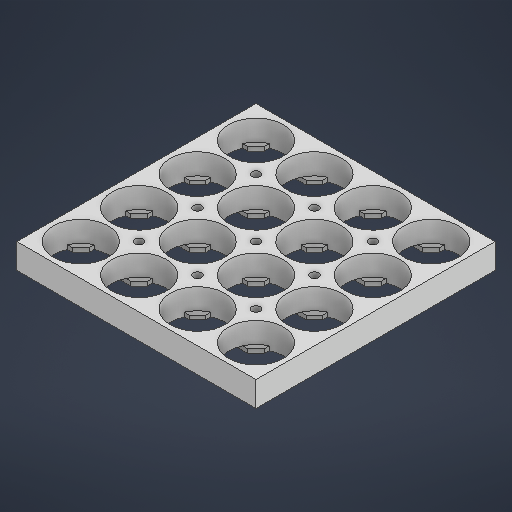
# Autodesk Inventor part: battery_pack_16s_rear
Saved by Autodesk Inventor 2026.1 (Build 301233000, 233)
## iProperties
Created: 2026-03-08
Part Number: battery_pack_16s_rear
Material: Generic
Document SubType Name: Modeling
Designer: aaron
Density: 1 g/cm^3
Appearance: Default
Author: aaron
Autodesk Inventor part; units mm, degrees
ref_plane "YZ Plane" through (0, 0, 0) normal (1, 0, 0) x (0, 1, 0)
ref_plane "XZ Plane" through (0, 0, 0) normal (0, 1, 0) x (-1, 0, 0)
ref_plane "XY Plane" through (0, 0, 0) normal (0, 0, 1) x (1, 0, 0)
sketch "Sketch1" plane through (0, 0, 0) normal (0, 1, 0) x (-1, 0, 0)
  circle A0 centre (10.0499, 9.6753) radius 13.1
  line L0 (10.0499, 9.6753) -> (10.0499, 15.7412)
  line L1 (10.0499, 9.6753) -> (16.8689, 9.6753)
  circle A1 centre (10.0499, 37.6753) radius 13.1
  circle A2 centre (10.0499, 65.6753) radius 13.1
  circle A3 centre (10.0499, 93.6753) radius 13.1
  circle A4 centre (38.0499, 9.6753) radius 13.1
  circle A5 centre (38.0499, 37.6753) radius 13.1
  circle A6 centre (38.0499, 65.6753) radius 13.1
  circle A7 centre (38.0499, 93.6753) radius 13.1
  circle A8 centre (66.0499, 9.6753) radius 13.1
  circle A9 centre (66.0499, 37.6753) radius 13.1
  circle A10 centre (66.0499, 65.6753) radius 13.1
  circle A11 centre (66.0499, 93.6753) radius 13.1
  circle A12 centre (94.0499, 9.6753) radius 13.1
  circle A13 centre (94.0499, 37.6753) radius 13.1
  circle A14 centre (94.0499, 65.6753) radius 13.1
  circle A15 centre (94.0499, 93.6753) radius 13.1
  line L2 (109.3499, 108.9753) -> (-5.2501, 108.9753)
  line L3 (-5.2501, 108.9753) -> (-5.2501, -5.6247)
  line L4 (-5.2501, -5.6247) -> (109.3499, -5.6247)
  line L5 (109.3499, -5.6247) -> (109.3499, 108.9753)
  point P0 (0, 0)
  dimension "d0" = 26.2
  dimension "d3" = 28
  dimension "d6" = 28
  dimension "d9" = 15.3
  dimension "d10" = 15.3
  dimension "d11" = 15.3
  dimension "d12" = 15.3
  constraints: 16 centre point, 12 end point, 3 horizontal, 2 parallel, 2 vertical, 1 perpendicular, 30 other
  measures "d0" diameter of A0
  measures "d3" distance of L0.start A1.centre
  measures "d6" distance of L0.start A4.centre
  measures "d9" distance from line of L5 A15.centre
  measures "d10" distance from line of L3 A3.centre
  measures "d11" distance from line of L2 A15.centre
  measures "d12" distance from line of L4 A12.centre
extrude "Extrusion1" add sketch "Sketch1" along normal blind 10
sketch "Sketch2" plane through (0, 0, 0) normal (0, -1, 0) x (1, 0, 0)
  line L0 (-109.3499, 108.9753) -> (5.2501, 108.9753) projected
  line L1 (5.2501, 108.9753) -> (5.2501, -5.6247) projected
  line L2 (5.2501, -5.6247) -> (-109.3499, -5.6247) projected
  line L3 (-109.3499, -5.6247) -> (-109.3499, 108.9753) projected
  circle A0 centre (-10.0499, 93.6753) radius 13.1 projected
  circle A1 centre (-10.0499, 9.6753) radius 13.1 projected
  line L4 (8.4501, 116.1753) -> (-0.5499, 116.1753)
  line L5 (-4.5499, 112.1753) -> (-4.5499, 103.1753)
  line L6 (-0.5499, 99.1753) -> (8.4501, 99.1753)
  line L7 (12.4501, 103.1753) -> (12.4501, 112.1753)
  line L8 (-10.0499, 93.6753) -> (15.9741, 93.6753)
  line L9 (-10.0499, 93.6753) -> (-10.0499, 119.9276)
  circle A2 centre (-38.0499, 93.6753) radius 13.1 projected
  circle A3 centre (-38.0499, 65.6753) radius 13.1 projected
  line L10 (-38.0499, 93.6753) -> (-38.0499, 65.6753)
  circle A4 centre (-66.0499, 65.6753) radius 13.1 projected
  line L11 (-38.0499, 65.6753) -> (-66.0499, 65.6753)
  line L12 (-4.5499, 103.1753) -> (-0.5499, 99.1753)
  line L13 (-0.5499, 116.1753) -> (-4.5499, 112.1753)
  line L14 (8.4501, 116.1753) -> (12.4501, 112.1753)
  line L15 (8.4501, 99.1753) -> (12.4501, 103.1753)
  line L16 (8.4501, 88.1753) -> (12.4501, 84.1753)
  line L17 (12.4501, 75.1753) -> (12.4501, 84.1753)
  line L18 (8.4501, 88.1753) -> (-0.5499, 88.1753)
  line L19 (-0.5499, 88.1753) -> (-4.5499, 84.1753)
  line L20 (-4.5499, 84.1753) -> (-4.5499, 75.1753)
  line L21 (-4.5499, 75.1753) -> (-0.5499, 71.1753)
  line L22 (-0.5499, 71.1753) -> (8.4501, 71.1753)
  line L23 (8.4501, 71.1753) -> (12.4501, 75.1753)
  line L24 (8.4501, 60.1753) -> (12.4501, 56.1753)
  line L25 (12.4501, 47.1753) -> (12.4501, 56.1753)
  line L26 (8.4501, 60.1753) -> (-0.5499, 60.1753)
  line L27 (-0.5499, 60.1753) -> (-4.5499, 56.1753)
  line L28 (-4.5499, 56.1753) -> (-4.5499, 47.1753)
  line L29 (-4.5499, 47.1753) -> (-0.5499, 43.1753)
  line L30 (-0.5499, 43.1753) -> (8.4501, 43.1753)
  line L31 (8.4501, 43.1753) -> (12.4501, 47.1753)
  line L32 (8.4501, 32.1753) -> (12.4501, 28.1753)
  line L33 (12.4501, 19.1753) -> (12.4501, 28.1753)
  line L34 (8.4501, 32.1753) -> (-0.5499, 32.1753)
  line L35 (-0.5499, 32.1753) -> (-4.5499, 28.1753)
  line L36 (-4.5499, 28.1753) -> (-4.5499, 19.1753)
  line L37 (-4.5499, 19.1753) -> (-0.5499, 15.1753)
  line L38 (-0.5499, 15.1753) -> (8.4501, 15.1753)
  line L39 (8.4501, 15.1753) -> (12.4501, 19.1753)
  line L40 (8.4501, 4.1753) -> (12.4501, 0.1753)
  line L41 (12.4501, -8.8247) -> (12.4501, 0.1753)
  line L42 (8.4501, 4.1753) -> (-0.5499, 4.1753)
  line L43 (-0.5499, 4.1753) -> (-4.5499, 0.1753)
  line L44 (-4.5499, 0.1753) -> (-4.5499, -8.8247)
  line L45 (-4.5499, -8.8247) -> (-0.5499, -12.8247)
  line L46 (-0.5499, -12.8247) -> (8.4501, -12.8247)
  line L47 (8.4501, -12.8247) -> (12.4501, -8.8247)
  line L48 (-19.5499, 116.1753) -> (-15.5499, 112.1753)
  line L49 (-15.5499, 103.1753) -> (-15.5499, 112.1753)
  line L50 (-19.5499, 116.1753) -> (-28.5499, 116.1753)
  line L51 (-28.5499, 116.1753) -> (-32.5499, 112.1753)
  line L52 (-32.5499, 112.1753) -> (-32.5499, 103.1753)
  line L53 (-32.5499, 103.1753) -> (-28.5499, 99.1753)
  line L54 (-28.5499, 99.1753) -> (-19.5499, 99.1753)
  line L55 (-19.5499, 99.1753) -> (-15.5499, 103.1753)
  line L56 (-19.5499, 88.1753) -> (-15.5499, 84.1753)
  line L57 (-15.5499, 75.1753) -> (-15.5499, 84.1753)
  line L58 (-19.5499, 88.1753) -> (-28.5499, 88.1753)
  line L59 (-28.5499, 88.1753) -> (-32.5499, 84.1753)
  line L60 (-32.5499, 84.1753) -> (-32.5499, 75.1753)
  line L61 (-32.5499, 75.1753) -> (-28.5499, 71.1753)
  line L62 (-28.5499, 71.1753) -> (-19.5499, 71.1753)
  line L63 (-19.5499, 71.1753) -> (-15.5499, 75.1753)
  line L64 (-19.5499, 60.1753) -> (-15.5499, 56.1753)
  line L65 (-15.5499, 47.1753) -> (-15.5499, 56.1753)
  line L66 (-19.5499, 60.1753) -> (-28.5499, 60.1753)
  line L67 (-28.5499, 60.1753) -> (-32.5499, 56.1753)
  line L68 (-32.5499, 56.1753) -> (-32.5499, 47.1753)
  line L69 (-32.5499, 47.1753) -> (-28.5499, 43.1753)
  line L70 (-28.5499, 43.1753) -> (-19.5499, 43.1753)
  line L71 (-19.5499, 43.1753) -> (-15.5499, 47.1753)
  line L72 (-19.5499, 32.1753) -> (-15.5499, 28.1753)
  line L73 (-15.5499, 19.1753) -> (-15.5499, 28.1753)
  line L74 (-19.5499, 32.1753) -> (-28.5499, 32.1753)
  line L75 (-28.5499, 32.1753) -> (-32.5499, 28.1753)
  line L76 (-32.5499, 28.1753) -> (-32.5499, 19.1753)
  line L77 (-32.5499, 19.1753) -> (-28.5499, 15.1753)
  line L78 (-28.5499, 15.1753) -> (-19.5499, 15.1753)
  line L79 (-19.5499, 15.1753) -> (-15.5499, 19.1753)
  line L80 (-19.5499, 4.1753) -> (-15.5499, 0.1753)
  line L81 (-15.5499, -8.8247) -> (-15.5499, 0.1753)
  line L82 (-19.5499, 4.1753) -> (-28.5499, 4.1753)
  line L83 (-28.5499, 4.1753) -> (-32.5499, 0.1753)
  line L84 (-32.5499, 0.1753) -> (-32.5499, -8.8247)
  line L85 (-32.5499, -8.8247) -> (-28.5499, -12.8247)
  line L86 (-28.5499, -12.8247) -> (-19.5499, -12.8247)
  line L87 (-19.5499, -12.8247) -> (-15.5499, -8.8247)
  line L88 (-47.5499, 116.1753) -> (-43.5499, 112.1753)
  line L89 (-43.5499, 103.1753) -> (-43.5499, 112.1753)
  line L90 (-47.5499, 116.1753) -> (-56.5499, 116.1753)
  line L91 (-56.5499, 116.1753) -> (-60.5499, 112.1753)
  line L92 (-60.5499, 112.1753) -> (-60.5499, 103.1753)
  line L93 (-60.5499, 103.1753) -> (-56.5499, 99.1753)
  line L94 (-56.5499, 99.1753) -> (-47.5499, 99.1753)
  line L95 (-47.5499, 99.1753) -> (-43.5499, 103.1753)
  line L96 (-47.5499, 88.1753) -> (-43.5499, 84.1753)
  line L97 (-43.5499, 75.1753) -> (-43.5499, 84.1753)
  line L98 (-47.5499, 88.1753) -> (-56.5499, 88.1753)
  line L99 (-56.5499, 88.1753) -> (-60.5499, 84.1753)
  line L100 (-60.5499, 84.1753) -> (-60.5499, 75.1753)
  line L101 (-60.5499, 75.1753) -> (-56.5499, 71.1753)
  line L102 (-56.5499, 71.1753) -> (-47.5499, 71.1753)
  line L103 (-47.5499, 71.1753) -> (-43.5499, 75.1753)
  line L104 (-47.5499, 60.1753) -> (-43.5499, 56.1753)
  line L105 (-43.5499, 47.1753) -> (-43.5499, 56.1753)
  line L106 (-47.5499, 60.1753) -> (-56.5499, 60.1753)
  line L107 (-56.5499, 60.1753) -> (-60.5499, 56.1753)
  line L108 (-60.5499, 56.1753) -> (-60.5499, 47.1753)
  line L109 (-60.5499, 47.1753) -> (-56.5499, 43.1753)
  line L110 (-56.5499, 43.1753) -> (-47.5499, 43.1753)
  line L111 (-47.5499, 43.1753) -> (-43.5499, 47.1753)
  line L112 (-47.5499, 32.1753) -> (-43.5499, 28.1753)
  line L113 (-43.5499, 19.1753) -> (-43.5499, 28.1753)
  line L114 (-47.5499, 32.1753) -> (-56.5499, 32.1753)
  line L115 (-56.5499, 32.1753) -> (-60.5499, 28.1753)
  line L116 (-60.5499, 28.1753) -> (-60.5499, 19.1753)
  line L117 (-60.5499, 19.1753) -> (-56.5499, 15.1753)
  line L118 (-56.5499, 15.1753) -> (-47.5499, 15.1753)
  line L119 (-47.5499, 15.1753) -> (-43.5499, 19.1753)
  line L120 (-47.5499, 4.1753) -> (-43.5499, 0.1753)
  line L121 (-43.5499, -8.8247) -> (-43.5499, 0.1753)
  line L122 (-47.5499, 4.1753) -> (-56.5499, 4.1753)
  line L123 (-56.5499, 4.1753) -> (-60.5499, 0.1753)
  line L124 (-60.5499, 0.1753) -> (-60.5499, -8.8247)
  line L125 (-60.5499, -8.8247) -> (-56.5499, -12.8247)
  line L126 (-56.5499, -12.8247) -> (-47.5499, -12.8247)
  line L127 (-47.5499, -12.8247) -> (-43.5499, -8.8247)
  line L128 (-75.5499, 116.1753) -> (-71.5499, 112.1753)
  line L129 (-71.5499, 103.1753) -> (-71.5499, 112.1753)
  line L130 (-75.5499, 116.1753) -> (-84.5499, 116.1753)
  line L131 (-84.5499, 116.1753) -> (-88.5499, 112.1753)
  line L132 (-88.5499, 112.1753) -> (-88.5499, 103.1753)
  line L133 (-88.5499, 103.1753) -> (-84.5499, 99.1753)
  line L134 (-84.5499, 99.1753) -> (-75.5499, 99.1753)
  line L135 (-75.5499, 99.1753) -> (-71.5499, 103.1753)
  line L136 (-75.5499, 88.1753) -> (-71.5499, 84.1753)
  line L137 (-71.5499, 75.1753) -> (-71.5499, 84.1753)
  line L138 (-75.5499, 88.1753) -> (-84.5499, 88.1753)
  line L139 (-84.5499, 88.1753) -> (-88.5499, 84.1753)
  line L140 (-88.5499, 84.1753) -> (-88.5499, 75.1753)
  line L141 (-88.5499, 75.1753) -> (-84.5499, 71.1753)
  line L142 (-84.5499, 71.1753) -> (-75.5499, 71.1753)
  line L143 (-75.5499, 71.1753) -> (-71.5499, 75.1753)
  line L144 (-75.5499, 60.1753) -> (-71.5499, 56.1753)
  line L145 (-71.5499, 47.1753) -> (-71.5499, 56.1753)
  line L146 (-75.5499, 60.1753) -> (-84.5499, 60.1753)
  line L147 (-84.5499, 60.1753) -> (-88.5499, 56.1753)
  line L148 (-88.5499, 56.1753) -> (-88.5499, 47.1753)
  line L149 (-88.5499, 47.1753) -> (-84.5499, 43.1753)
  line L150 (-84.5499, 43.1753) -> (-75.5499, 43.1753)
  line L151 (-75.5499, 43.1753) -> (-71.5499, 47.1753)
  line L152 (-75.5499, 32.1753) -> (-71.5499, 28.1753)
  line L153 (-71.5499, 19.1753) -> (-71.5499, 28.1753)
  line L154 (-75.5499, 32.1753) -> (-84.5499, 32.1753)
  line L155 (-84.5499, 32.1753) -> (-88.5499, 28.1753)
  line L156 (-88.5499, 28.1753) -> (-88.5499, 19.1753)
  line L157 (-88.5499, 19.1753) -> (-84.5499, 15.1753)
  line L158 (-84.5499, 15.1753) -> (-75.5499, 15.1753)
  line L159 (-75.5499, 15.1753) -> (-71.5499, 19.1753)
  line L160 (-75.5499, 4.1753) -> (-71.5499, 0.1753)
  line L161 (-71.5499, -8.8247) -> (-71.5499, 0.1753)
  line L162 (-75.5499, 4.1753) -> (-84.5499, 4.1753)
  line L163 (-84.5499, 4.1753) -> (-88.5499, 0.1753)
  line L164 (-88.5499, 0.1753) -> (-88.5499, -8.8247)
  line L165 (-88.5499, -8.8247) -> (-84.5499, -12.8247)
  line L166 (-84.5499, -12.8247) -> (-75.5499, -12.8247)
  line L167 (-75.5499, -12.8247) -> (-71.5499, -8.8247)
  line L168 (-103.5499, 116.1753) -> (-99.5499, 112.1753)
  line L169 (-99.5499, 103.1753) -> (-99.5499, 112.1753)
  line L170 (-103.5499, 116.1753) -> (-112.5499, 116.1753)
  line L171 (-112.5499, 116.1753) -> (-116.5499, 112.1753)
  line L172 (-116.5499, 112.1753) -> (-116.5499, 103.1753)
  line L173 (-116.5499, 103.1753) -> (-112.5499, 99.1753)
  line L174 (-112.5499, 99.1753) -> (-103.5499, 99.1753)
  line L175 (-103.5499, 99.1753) -> (-99.5499, 103.1753)
  line L176 (-103.5499, 88.1753) -> (-99.5499, 84.1753)
  line L177 (-99.5499, 75.1753) -> (-99.5499, 84.1753)
  line L178 (-103.5499, 88.1753) -> (-112.5499, 88.1753)
  line L179 (-112.5499, 88.1753) -> (-116.5499, 84.1753)
  line L180 (-116.5499, 84.1753) -> (-116.5499, 75.1753)
  line L181 (-116.5499, 75.1753) -> (-112.5499, 71.1753)
  line L182 (-112.5499, 71.1753) -> (-103.5499, 71.1753)
  line L183 (-103.5499, 71.1753) -> (-99.5499, 75.1753)
  line L184 (-103.5499, 60.1753) -> (-99.5499, 56.1753)
  line L185 (-99.5499, 47.1753) -> (-99.5499, 56.1753)
  line L186 (-103.5499, 60.1753) -> (-112.5499, 60.1753)
  line L187 (-112.5499, 60.1753) -> (-116.5499, 56.1753)
  line L188 (-116.5499, 56.1753) -> (-116.5499, 47.1753)
  line L189 (-116.5499, 47.1753) -> (-112.5499, 43.1753)
  line L190 (-112.5499, 43.1753) -> (-103.5499, 43.1753)
  line L191 (-103.5499, 43.1753) -> (-99.5499, 47.1753)
  line L192 (-103.5499, 32.1753) -> (-99.5499, 28.1753)
  line L193 (-99.5499, 19.1753) -> (-99.5499, 28.1753)
  line L194 (-103.5499, 32.1753) -> (-112.5499, 32.1753)
  line L195 (-112.5499, 32.1753) -> (-116.5499, 28.1753)
  line L196 (-116.5499, 28.1753) -> (-116.5499, 19.1753)
  line L197 (-116.5499, 19.1753) -> (-112.5499, 15.1753)
  line L198 (-112.5499, 15.1753) -> (-103.5499, 15.1753)
  line L199 (-103.5499, 15.1753) -> (-99.5499, 19.1753)
  line L200 (-103.5499, 4.1753) -> (-99.5499, 0.1753)
  line L201 (-99.5499, -8.8247) -> (-99.5499, 0.1753)
  line L202 (-103.5499, 4.1753) -> (-112.5499, 4.1753)
  line L203 (-112.5499, 4.1753) -> (-116.5499, 0.1753)
  line L204 (-116.5499, 0.1753) -> (-116.5499, -8.8247)
  line L205 (-116.5499, -8.8247) -> (-112.5499, -12.8247)
  line L206 (-112.5499, -12.8247) -> (-103.5499, -12.8247)
  line L207 (-103.5499, -12.8247) -> (-99.5499, -8.8247)
  circle A5 centre (-94.0499, 9.6753) radius 13.1 projected
  circle A6 centre (-94.0499, 37.6753) radius 13.1 projected
  circle A7 centre (-94.0499, 65.6753) radius 13.1 projected
  circle A8 centre (-94.0499, 93.6753) radius 13.1 projected
  circle A9 centre (-66.0499, 93.6753) radius 13.1 projected
  circle A10 centre (-66.0499, 37.6753) radius 13.1 projected
  circle A11 centre (-38.0499, 37.6753) radius 13.1 projected
  circle A12 centre (-66.0499, 9.6753) radius 13.1 projected
  circle A13 centre (-38.0499, 9.6753) radius 13.1 projected
  circle A14 centre (-10.0499, 37.6753) radius 13.1 projected
  circle A15 centre (-10.0499, 65.6753) radius 13.1 projected
  point P0 (12.4501, 116.1753)
  point P1 (-4.5499, 99.1753)
  point P2 (-4.5499, 116.1753)
  point P3 (12.4501, 99.1753)
  point P4 (-71.5499, -5.6247)
  point P5 (-77.9394, 4.1753)
  point P6 (-77.9394, 15.1753)
  point P7 (-71.5499, 21.5648)
  point P8 (-60.5499, 21.5648)
  point P9 (-54.1604, 15.1753)
  point P10 (-54.1604, 4.1753)
  point P11 (-60.5499, -5.6247)
  point P12 (1.8396, 99.1753)
  point P13 (1.8396, 88.1753)
  point P14 (-4.5499, 81.7858)
  point P15 (-15.5499, 81.7858)
  point P16 (-21.9394, 88.1753)
  point P17 (-21.9394, 99.1753)
  point P18 (-15.5499, 105.5648)
  point P19 (-4.5499, 105.5648)
  point P20 (1.8396, 4.1753)
  point P21 (-4.5499, -2.2142)
  point P22 (-15.5499, -2.2142)
  point P23 (-21.9394, 4.1753)
  point P24 (-21.9394, 15.1753)
  point P25 (-15.5499, 21.5648)
  point P26 (-4.5499, 21.5648)
  point P27 (1.8396, 15.1753)
  point P28 (-26.1604, 99.1753)
  point P29 (-26.1604, 88.1753)
  point P30 (-32.5499, 81.7858)
  point P31 (-43.5499, 81.7858)
  point P32 (-49.9394, 88.1753)
  point P33 (-49.9394, 99.1753)
  point P34 (-43.5499, 105.5648)
  point P35 (-32.5499, 105.5648)
  point P36 (-32.5499, 77.5648)
  point P37 (-26.1604, 71.1753)
  point P38 (-26.1604, 60.1753)
  point P39 (-32.5499, 53.7858)
  point P40 (-43.5499, 53.7858)
  point P41 (-49.9394, 60.1753)
  point P42 (-49.9394, 71.1753)
  point P43 (-43.5499, 77.5648)
  point P44 (-54.1604, 60.1753)
  point P45 (-60.5499, 53.7858)
  point P46 (-71.5499, 53.7858)
  point P47 (-77.9394, 60.1753)
  point P48 (-77.9394, 71.1753)
  point P49 (-71.5499, 77.5648)
  point P50 (-60.5499, 77.5648)
  point P51 (-54.1604, 71.1753)
  point P52 (-99.5499, -2.2142)
  point P53 (-105.9394, 4.1753)
  point P54 (-105.9394, 15.1753)
  point P55 (-99.5499, 21.5648)
  point P56 (-88.5499, 21.5648)
  point P57 (-82.1604, 15.1753)
  point P58 (-82.1604, 4.1753)
  point P59 (-88.5499, -2.2142)
  point P60 (-99.5499, 25.7858)
  point P61 (-105.9394, 32.1753)
  point P62 (-105.9394, 43.1753)
  point P63 (-99.5499, 49.5648)
  point P64 (-88.5499, 49.5648)
  point P65 (-82.1604, 43.1753)
  point P66 (-82.1604, 32.1753)
  point P67 (-88.5499, 25.7858)
  point P68 (-99.5499, 105.5648)
  point P69 (-88.5499, 105.5648)
  point P70 (-82.1604, 99.1753)
  point P71 (-82.1604, 88.1753)
  point P72 (-88.5499, 81.7858)
  point P73 (-99.5499, 81.7858)
  point P74 (-105.9394, 88.1753)
  point P75 (-105.9394, 99.1753)
  point P76 (-54.1604, 99.1753)
  point P77 (-54.1604, 88.1753)
  point P78 (-60.5499, 81.7858)
  point P79 (-71.5499, 81.7858)
  point P80 (-77.9394, 88.1753)
  point P81 (-77.9394, 99.1753)
  point P82 (-71.5499, 105.5648)
  point P83 (-60.5499, 105.5648)
  point P84 (-43.5499, 21.5648)
  point P85 (-32.5499, 21.5648)
  point P86 (-26.1604, 15.1753)
  point P87 (-26.1604, 4.1753)
  point P88 (-32.5499, -2.2142)
  point P89 (-43.5499, -2.2142)
  point P90 (-49.9394, 4.1753)
  point P91 (-49.9394, 15.1753)
  point P92 (1.8396, 71.1753)
  point P93 (1.8396, 60.1753)
  point P94 (-4.5499, 53.7858)
  point P95 (-15.5499, 53.7858)
  point P96 (-21.9394, 60.1753)
  point P97 (-21.9394, 71.1753)
  point P98 (-15.5499, 77.5648)
  point P99 (-4.5499, 77.5648)
  point P100 (1.8396, 32.1753)
  point P101 (-4.5499, 25.7858)
  point P102 (-15.5499, 25.7858)
  point P103 (-21.9394, 32.1753)
  point P104 (-21.9394, 43.1753)
  point P105 (-15.5499, 49.5648)
  point P106 (-4.5499, 49.5648)
  point P107 (1.8396, 43.1753)
  point P108 (-49.9394, 43.1753)
  point P109 (-43.5499, 49.5648)
  point P110 (-32.5499, 49.5648)
  point P111 (-26.1604, 43.1753)
  point P112 (-26.1604, 32.1753)
  point P113 (-32.5499, 25.7858)
  point P114 (-43.5499, 25.7858)
  point P115 (-49.9394, 32.1753)
  point P116 (-77.9394, 43.1753)
  point P117 (-71.5499, 49.5648)
  point P118 (-60.5499, 49.5648)
  point P119 (-54.1604, 43.1753)
  point P120 (-54.1604, 32.1753)
  point P121 (-60.5499, 25.7858)
  point P122 (-71.5499, 25.7858)
  point P123 (-77.9394, 32.1753)
  point P124 (-99.5499, 53.7858)
  point P125 (-105.9394, 60.1753)
  point P126 (-105.9394, 71.1753)
  point P127 (-99.5499, 77.5648)
  point P128 (-88.5499, 77.5648)
  point P129 (-82.1604, 71.1753)
  point P130 (-82.1604, 60.1753)
  point P131 (-88.5499, 53.7858)
  point P132 (-60.5499, -2.2142)
  point P133 (-71.5499, -2.2142)
  point P134 (5.2501, 99.1753)
  point P135 (-4.5499, 108.9753)
  point P136 (5.2501, 71.1753)
  point P137 (5.2501, 88.1753)
  point P138 (-109.3499, 4.1753)
  point P139 (-99.5499, -5.6247)
  point P140 (-109.3499, 32.1753)
  point P141 (-109.3499, 15.1753)
  point P142 (-109.3499, 60.1753)
  point P143 (-109.3499, 43.1753)
  point P144 (-99.5499, 108.9753)
  point P145 (-109.3499, 99.1753)
  point P146 (-109.3499, 88.1753)
  point P147 (-109.3499, 71.1753)
  point P148 (-88.5499, -5.6247)
  point P149 (-71.5499, 108.9753)
  point P150 (-88.5499, 108.9753)
  point P151 (-43.5499, -5.6247)
  point P152 (-43.5499, 108.9753)
  point P153 (-60.5499, 108.9753)
  point P154 (-4.5499, -5.6247)
  point P155 (5.2501, 4.1753)
  point P156 (-32.5499, -5.6247)
  point P157 (-15.5499, -5.6247)
  point P158 (5.2501, 15.1753)
  point P159 (5.2501, 32.1753)
  point P160 (5.2501, 43.1753)
  point P161 (5.2501, 60.1753)
  point P162 (-15.5499, 108.9753)
  point P163 (-32.5499, 108.9753)
  dimension "d19" = 17
  dimension "d20" = 17
  dimension "d21" = 5.5
  dimension "d22" = 28
  dimension "d23" = 5.5
  dimension "d24" = 4
  dimension "d25" = 4
  dimension "d26" = 4
  dimension "d27" = 4
  dimension "d28" = 4
  dimension "d29" = 4
  dimension "d30" = 4
  dimension "d31" = 4
  dimension "d34" = 28
  dimension "d37" = 28
  constraints: 408 end point, 8 point on line, 3 horizontal, 3 vertical, 2 parallel, 2 perpendicular, 384 other
  measures "d19" distance of point (12.45, 116.175) point (-4.55, 116.175)
  measures "d20" distance of point (12.45, 99.175) point (12.45, 116.175)
  measures "d21" distance between parallel lines of L8 L6
  measures "d22" distance of L10.start L10.end
  measures "d23" distance between parallel lines of L9 L5
  measures "d24" distance of L5.end point (-4.55, 99.175)
  measures "d25" distance of L6.start point (-4.55, 99.175)
  measures "d26" distance of L4.end point (-4.55, 116.175)
  measures "d27" distance of L5.start point (-4.55, 116.175)
  measures "d28" distance of L4.start point (12.45, 116.175)
  measures "d29" distance of L7.end point (12.45, 116.175)
  measures "d30" distance of L6.end point (12.45, 99.175)
  measures "d31" distance of L7.start point (12.45, 99.175)
  measures "d34" distance of L4.start L16.start
  measures "d37" distance of L4.start L48.start
extrude "Extrusion2" add sketch "Sketch2" along normal blind 2 contours L0 L169 A8 L174 L3 | L0 L132 A8 L169 | L174 A8 L178 L3 | L0 L129 A9 L134 A8 L132 | L169 L175 L174 A8 | L178 A8 L177 A7 L182 L3 | L0 L92 A9 L129 | A8 L134 L133 L132 | L182 A7 L186 L3 | L178 L176 L177 A8 | L0 L89 A2 L94 A9 L92 | L129 L135 L134 A9 | L186 A7 L185 A6 L190 L3 | A7 L177 L183 L182 | A8 L140 A7 L177 | L0 L52 A2 L89 | A9 L94 L93 L92 | L190 A6 L194 L3 | L186 L184 L185 A7 | A8 L138 A9 L137 A4 L142 A7 L140 | L140 L139 L138 A8 | L0 L49 A0 L54 A2 L52 | L89 L95 L94 A2 | L94 A2 L98 A9 | L138 L136 L137 A9 | L194 A6 L193 A5 L198 L3 | A6 L185 L191 L190 | A7 L148 A6 L185 | A7 L142 L141 L140 | L0 L9 A0 L49 | A2 L54 L53 L52 | A9 L100 A4 L137 | L198 A5 L202 L3 | L194 L192 L193 A6 | A7 L146 A4 L145 A10 L150 A6 L148 | L148 L147 L146 A7 | L0 L5 A0 L9 | L49 L55 L54 A0 | L98 L96 L97 A2 | A2 L97 A3 L102 A4 L100 A9 L98 | A9 L100 L99 L98 | L137 L143 L142 A4 | L202 A5 L201 L2 L3 | A5 L193 L199 L198 | A6 L156 A5 L193 | A6 L150 L149 L148 | L0 L1 L6 A0 L5 | A2 L10 A3 L97 | A4 L102 L101 L100 | L202 L200 L201 A5 | A6 L154 A10 L153 A12 L158 A5 L156 | L156 L155 L154 A6 | L146 L144 L145 A4 | A0 L6 L12 L5 | L58 L56 L57 A0 | A0 L57 A15 L62 A3 L60 A2 L58 | A2 L60 L59 L58 | A2 L60 A3 L10 | L97 L103 L102 A3 | L102 A3 L11 A4 | L201 A5 L164 L2 | A5 L158 L157 L156 | A10 L145 L151 L150 | A4 L108 A10 L145 | L1 L8 A0 L6 | L8 L1 L18 A0 | A0 L20 A15 L57 | L11 A3 L106 A4 | L164 A5 L162 A12 L161 L2 | L164 L163 L162 A5 | L154 L152 L153 A10 | L108 L107 L106 A4 | A4 L106 A3 L105 A11 L110 A10 L108 | L18 L1 L22 A15 L20 A0 | A0 L20 L19 L18 | L57 L63 L62 A15 | A3 L62 L61 L60 | L161 A12 L124 L2 | A12 L153 L159 L158 | A10 L116 A12 L153 | A10 L110 L109 L108 | A15 L22 L21 L20 | L106 L104 L105 A3 | L124 A12 L122 A13 L121 L2 | A12 L162 L160 L161 | A10 L114 A11 L113 A13 L118 A12 L116 | L116 L115 L114 A10 | L110 A11 L114 A10 | L1 L26 A15 L22 | A15 L65 A14 L70 A11 L68 A3 L66 | L66 L64 L65 A15 | A3 L68 A11 L105 | L121 A13 L84 L2 | L124 L123 L122 A12 | A12 L118 L117 L116 | A11 L105 L111 L110 | L1 L30 A14 L28 A15 L26 | A3 L68 L67 L66 | A15 L28 A14 L65 | L84 A13 L82 A1 L81 L2 | A13 L122 L120 L121 | A12 L118 A13 L122 | L114 L112 L113 A11 | L1 L34 A14 L30 | A15 L28 L27 L26 | L65 L71 L70 A14 | A11 L70 L69 L68 | L81 A1 L44 L2 | L84 L83 L82 A13 | A13 L113 L119 L118 | A11 L76 A13 L113 | L1 L38 A1 L36 A14 L34 | L30 L29 L28 A14 | L44 A1 L42 L1 L2 | A1 L82 L80 L81 | A11 L74 A14 L73 A1 L78 A13 L76 | L76 L75 L74 A11 | L1 L42 A1 L38 | A14 L36 L35 L34 | L74 L72 L73 A14 | L44 L43 L42 A1 | A13 L78 L77 L76 | L38 L37 L36 A1 | L36 A1 L73 A14 | A1 L73 L79 L78
sketch "Sketch3" plane through (0, -2, 0) normal (0, -1, 0) x (1, 0, 0)
  arc A0 (-33.2499, 78.2648) -> (-44.2499, 78.2648) centre (-38.7499, 66.3753) ccw projected
  circle A1 centre (-38.0499, 37.6753) radius 13.1 projected
  line L0 (-38.7499, 66.3753) -> (-38.7499, 37.6753)
  circle A2 centre (-66.0499, 37.6753) radius 13.1 projected
  line L1 (-38.0499, 37.6753) -> (-66.0499, 37.6753)
  circle A3 centre (-24.0499, 79.6753) radius 2
  line L2 (-15.5499, 75.1753) -> (-15.5499, 84.1753) projected
  line L3 (-32.5499, 84.1753) -> (-32.5499, 75.1753) projected
  line L4 (-19.5499, 88.1753) -> (-28.5499, 88.1753) projected
  circle A4 centre (-24.0499, 51.6753) radius 2
  circle A5 centre (-24.0499, 23.6753) radius 2
  circle A6 centre (-52.0499, 79.6753) radius 2
  circle A7 centre (-52.0499, 51.6753) radius 2
  circle A8 centre (-52.0499, 23.6753) radius 2
  circle A9 centre (-80.0499, 79.6753) radius 2
  circle A10 centre (-80.0499, 51.6753) radius 2
  circle A11 centre (-80.0499, 23.6753) radius 2
  point P0 (0, 0)
  point P1 (-32.5499, 75.1753)
  point P2 (-32.5499, 79.6753)
  dimension "d42" = 17
  dimension "d43" = 8.5
  dimension "d44" = 8.5
  dimension "d45" = 4
  dimension "d48" = 28
  dimension "d51" = 28
  constraints: 9 centre point, 4 end point, 2 vertical, 1 horizontal, 1 perpendicular, 18 other
  measures "d43" distance of point (-32.55, 79.675) A3.centre
  measures "d44" distance from line of L4 A3.centre
  measures "d45" diameter of A3
  measures "d48" distance of A3.centre A4.centre
  measures "d51" distance of A3.centre A6.centre
extrude "Extrusion3" cut sketch "Sketch3" against normal through all contours A3 | A4 | A5 | A6 | A7 | A8 | A9 | A10 | A11
equation "\"d10\" = d9"
equation "\"d11\" = d9"
equation "\"d12\" = d9"
equation "\"d20\" = d19"
equation "\"d21\" = -0.5 * d20 + 0.5 * d22"
equation "\"d23\" = d21"
equation "\"d25\" = d24"
equation "\"d26\" = d24"
equation "\"d27\" = d26"
equation "\"d28\" = d24"
equation "\"d29\" = d28"
equation "\"d30\" = d24"
equation "\"d31\" = d30"
body "Solid1"
